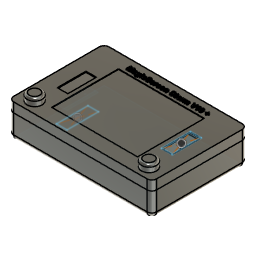
Coffret_telecran_nucleo_sharp (Autodesk Fusion 360 design; units mm, degrees)
Autodesk Fusion 360 part; units mm, degrees
(part 1 of 2)
sketch "Esquisse1" plane through (0, 0, 0) normal (0, 0, 1) x (1, 0, 0)
  line L0 (150, 100) -> (-150, 100)
  line L1 (-150, 100) -> (-150, -100)
  line L2 (-150, -100) -> (150, -100)
  line L3 (150, -100) -> (150, 100)
  line L4 (150, 100) -> (-150, -100) construction
  line L5 (-150, 100) -> (150, -100) construction
  dimension "d1" = 300
  dimension "d2" = 200
  constraint horizontal L0
  constraint perpendicular L0 L1
  constraint parallel L0 L2
  constraint parallel L1 L3
  constraint coincident L4 origin
  constraint coincident L5 origin
  measures "d1" distance of L0.start L0.end
  measures "d2" distance of L0.end L1.end
extrude "Extrusion1" add sketch "Esquisse1" along normal blind 50 makes body 1
extrude "Extrusion2" add 1 faces at (50, -33.3333, 50) along direction (0, 0, 1) blind 20 separate body on bodies 1 makes body 2
fillet "Congé1" radius 10 8 edges at (150, -100, 25) (150, 100, 25) (-150, 100, 25) (-150, -100, 25) (150, -100, 60) (150, 100, 60) (-150, 100, 60) (-150, -100, 60) on bodies 1 2
fillet "Congé2" radius 10 1 faces at (46.6667, -33.3333, 0) on bodies 1
shell "Coque1" thickness 5 removed faces 1 at (46.6667, -33.3333, 50) on bodies 1
hole "Perçage1" at (5.1249, 100, 27.601) direction (0, -1, 0) diameter 20 depth 30 tip angle 118 bodies 1
sketch "Esquisse2" plane through (0, 0, 5) normal (0, 0, 1) x (-1, 0, 0)
  line L0 (140, -90) -> (140, 90)
  line L1 (140, 90) -> (-140, 90)
  line L2 (-140, 90) -> (-140, -90)
  line L3 (-140, -90) -> (140, -90)
  line L4 (60, -50.203) -> (-60, -50.203)
  line L5 (-60, -50.203) -> (-60, 50.203)
  line L6 (-60, 50.203) -> (60, 50.203)
  line L7 (60, 50.203) -> (60, -50.203)
  line L8 (60, -50.203) -> (-60, 50.203) construction
  line L9 (-60, -50.203) -> (60, 50.203) construction
  dimension "d15" = 120
  dimension "d16" = 100.406
  constraint horizontal L4
  constraint perpendicular L4 L5
  constraint parallel L4 L6
  constraint parallel L5 L7
  constraint coincident L8 origin
  constraint coincident L9 origin
  measures "d15" distance of L4.start L4.end
  measures "d16" distance of L4.start L6.end
extrude "Extrusion3" add sketch "Esquisse2" along normal blind 35 separate body contours L4 L5 L6 L7 makes body 3
shell "Coque2" thickness 2 removed faces 1 at (-20, 16.7343, 40) on bodies 3
hole "Perçage2" at (-60, 2.6832, 20.4702) direction (1, 0, 0) diameter 20 depth 30 tip angle 118 bodies 3
hole "Perçage3" at (4.0962, 50.203, 25.4358) direction (0, -1, 0) diameter 20 depth 30 tip angle 118 bodies 3
hole "Perçage4" at (60, 1.6292, 22.5117) direction (-1, 0, 0) diameter 20 depth 3 tip angle 118 bodies 3
sketch "Esquisse3" plane through (0, 0, 5) normal (0, 0, 1) x (-1, 0, 0)
  line L0 (140, -90) -> (140, 90)
  line L1 (140, 90) -> (-140, 90)
  line L2 (-140, 90) -> (-140, -90)
  line L3 (-140, -90) -> (140, -90)
  line L4 (98, -36) -> (120, -36)
  line L5 (120, -36) -> (120, 30)
  line L6 (120, 30) -> (98, 30)
  line L7 (98, 30) -> (98, -36)
  line L8 (98, -36) -> (120, 30) construction
  line L9 (120, -36) -> (98, 30) construction
  point P0 (109, -3)
  point P1 (109, -3)
  dimension "d29" = 22
  constraint horizontal L4
  constraint perpendicular L4 L5
  constraint parallel L4 L6
  constraint parallel L5 L7
  constraint coincident L8 P1
  constraint coincident L9 P1
  measures "d29" distance of L5.end L6.end
extrude "Extrusion4" add sketch "Esquisse3" along normal blind 35 separate body contours L4 L5 L6 L7 makes body 4
hole "Perçage5" at (-109.1164, 19.6005, 40) direction (0, 0, -1) diameter 3.2 depth 3 tip angle 118 bodies 4
sketch "Esquisse4" plane through (0, 0, 40) normal (0, 0, 1) x (-1, 0, 0)
  circle A0 centre (109.1164, -19.6005) radius 1.6
  line L0 (98, 30) -> (98, -36)
  line L1 (98, -36) -> (120, -36)
  line L2 (120, -36) -> (120, 30)
  line L3 (120, 30) -> (98, 30)
hole "Perçage6" at (-109.2628, -17.4891, 40) direction (0, 0, -1) diameter 3.2 depth 3 tip angle 118 bodies 4
copy_body "Copier/Coller des corps2" bodies 4 makes body 5
move_body "Déplacer2" bodies 5 to x (1, 0, 0) y (0, 1, 0) z (0, 0, 1) at (220, 0, 0)
sketch "Esquisse5" plane through (0, 0, 70) normal (0, 0, 1) x (-1, 0, 0)
  arc A0 (150, 90) -> (140, 100) centre (140, 90) ccw
  line L0 (140, 100) -> (-140, 100)
  arc A1 (-140, 100) -> (-150, 90) centre (-140, 90) ccw
  line L1 (-150, 90) -> (-150, -90)
  arc A2 (-150, -90) -> (-140, -100) centre (-140, -90) ccw
  line L2 (-140, -100) -> (140, -100)
  arc A3 (140, -100) -> (150, -90) centre (140, -90) ccw
  line L3 (150, -90) -> (150, 90)
  line L4 (119.4908, 29.5506) -> (97.4908, 29.5506)
  line L5 (97.4908, 29.5506) -> (97.4908, -30.4494)
  line L6 (97.4908, -30.4494) -> (119.4908, -30.4494)
  line L7 (119.4908, -30.4494) -> (119.4908, 29.5506)
  line L8 (119.4908, 29.5506) -> (97.4908, -30.4494) construction
  line L9 (97.4908, 29.5506) -> (119.4908, -30.4494) construction
  point P0 (108.4908, -0.4494)
  dimension "d45" = 60
  dimension "d46" = 22
  constraint horizontal L4
  constraint perpendicular L4 L5
  constraint parallel L4 L6
  constraint parallel L5 L7
  constraint coincident L8 P0
  constraint coincident L9 P0
  measures "d45" distance of L4.end L5.end
  measures "d46" distance of L5.end L6.end
shell "Coque3" thickness 2 removed faces 1 at (46.6667, -33.3333, 50) on bodies 2
extrude "Extrusion5" cut sketch "Esquisse5" along normal blind 10 contours L4 L5 L6 L7 bodies 2
sketch "Esquisse6" plane through (0, 0, 70) normal (0, 0, 1) x (-1, 0, 0)
  line L0 (-100.2184, 29.3056) -> (-122.2184, 29.3056)
  line L1 (-122.2184, 29.3056) -> (-122.2184, -30.8073)
  line L2 (-122.2184, -30.8073) -> (-100.2184, -30.8073)
  line L3 (-100.2184, -30.8073) -> (-100.2184, 29.3056)
  line L4 (-100.2184, 29.3056) -> (-122.2184, -30.8073) construction
  line L5 (-122.2184, 29.3056) -> (-100.2184, -30.8073) construction
  point P0 (-111.2184, -0.7508)
  dimension "d51" = 60.1129
  dimension "d52" = 22
  constraint horizontal L0
  constraint perpendicular L0 L1
  constraint parallel L0 L2
  constraint parallel L1 L3
  constraint coincident L4 P0
  constraint coincident L5 P0
  measures "d51" distance of L0.end L1.end
  measures "d52" distance of L1.end L2.end
extrude "Extrusion6" cut sketch "Esquisse6" along normal blind 10 bodies 2
sketch "Esquisse7" plane through (0, 0, 70) normal (0, 0, 1) x (-1, 0, 0)
  arc A0 (150, 90) -> (140, 100) centre (140, 90) ccw
  line L0 (140, 100) -> (-140, 100)
  arc A1 (-140, 100) -> (-150, 90) centre (-140, 90) ccw
  line L1 (-150, 90) -> (-150, -90)
  arc A2 (-150, -90) -> (-140, -100) centre (-140, -90) ccw
  line L2 (-140, -100) -> (140, -100)
  arc A3 (140, -100) -> (150, -90) centre (140, -90) ccw
  line L3 (150, -90) -> (150, 90)
  line L4 (86.8869, -41.1186) -> (-95.6253, -41.0435) construction
  line L5 (-95.6253, -41.0435) -> (-95.6437, -85.9278) construction
  line L6 (-95.6437, -85.9278) -> (86.8684, -86.0029) construction
  line L7 (86.8684, -86.0029) -> (86.8869, -41.1186) construction
  dimension "d55" = 10
  text T0 "MagicScreen Storm V10 +" font "Arial" height 10 bold align centre top in box 182.5122 x 44.8843 at (86.8869, -41.1186) x (-1, 0.000412) y (-0.000412, -1) spacing 1
sketch "Esquisse8" plane through (0, 0, 70) normal (0, 0, 1) x (-1, 0, 0)
  line L0 (90, -70) -> (-90, -70)
  line L1 (-90, -70) -> (-90, 70)
  line L2 (-90, 70) -> (90, 70)
  line L3 (90, 70) -> (90, -70)
  constraint horizontal L0
  constraint vertical L1
  constraint horizontal L2
  constraint vertical L3
extrude "Extrusion7" cut sketch "Esquisse8" against normal blind 1 bodies 2
sketch "Esquisse9" plane through (0, 0, 70) normal (0, 0, 1) x (-1, 0, 0)
  circle A0 centre (120.2726, 75.6782) radius 15.6949
extrude "Extrusion8" add sketch "Esquisse9" along normal blind 15 separate body makes body 6
fillet "Congé3" radius 5 1 edges at (-105.6398, -70.0027, 85) on bodies 6
copy_body "Copier/Coller des corps3" bodies 6 makes body 7
move_body "Déplacer3" bodies 7 to x (1, 0, 0) y (0, 1, 0) z (0, 0, 1) at (240, 0, 0)
extrude "Extrusion9" add sketch "Esquisse7" along normal blind 2 text T0 bodies 2
sketch "Esquisse10" plane through (0, 0, 50) normal (0, 0, 1) x (-1, 0, 0)
  arc A0 (145, 90) -> (140, 95) centre (140, 90) ccw
  line L0 (145, 90) -> (145, -90)
  arc A1 (140, -95) -> (145, -90) centre (140, -90) ccw
  line L1 (140, -95) -> (-140, -95)
  arc A2 (-145, -90) -> (-140, -95) centre (-140, -90) ccw
  line L2 (-145, -90) -> (-145, 90)
  arc A3 (-140, 95) -> (-145, 90) centre (-140, 90) ccw
  line L3 (-140, 95) -> (140, 95)
  arc A4 (150, 90) -> (140, 100) centre (140, 90) ccw
  line L4 (140, 100) -> (-140, 100)
  arc A5 (-140, 100) -> (-150, 90) centre (-140, 90) ccw
  line L5 (-150, 90) -> (-150, -90)
  arc A6 (-150, -90) -> (-140, -100) centre (-140, -90) ccw
  line L6 (-140, -100) -> (140, -100)
  arc A7 (140, -100) -> (150, -90) centre (140, -90) ccw
  line L7 (150, -90) -> (150, 90)
  arc A8 (148, 90) -> (140, 98) centre (140, 90) ccw
  line L8 (140, 98) -> (-140, 98)
  arc A9 (-140, 98) -> (-148, 90) centre (-140, 90) ccw
  line L9 (-148, 90) -> (-148, -90)
  arc A10 (-148, -90) -> (-140, -98) centre (-140, -90) ccw
  line L10 (-140, -98) -> (140, -98)
  arc A11 (140, -98) -> (148, -90) centre (140, -90) ccw
  line L11 (148, -90) -> (148, 90)
  arc A12 (150, 90) -> (140, 100) centre (140, 90) ccw
  line L12 (150, 90) -> (150, -90)
  arc A13 (140, -100) -> (150, -90) centre (140, -90) ccw
  line L13 (140, -100) -> (-140, -100)
  arc A14 (-150, -90) -> (-140, -100) centre (-140, -90) ccw
  line L14 (-150, -90) -> (-150, 90)
  arc A15 (-140, 100) -> (-150, 90) centre (-140, 90) ccw
  line L15 (-140, 100) -> (140, 100)
extrude "Extrusion10" add sketch "Esquisse10" along normal blind 5 contours A8 L8 A9 L9 A10 L10 A11 L11 bodies 1
extrude "Extrusion12" cut sketch "Esquisse6" against normal blind 2 bodies 2
sketch "Esquisse11" plane through (0, 0, 70) normal (0, 0, 1) x (-1, 0, 0)
  line L0 (-122.2184, 29.3056) -> (-100.2184, 29.3056)
  line L1 (-100.2184, 29.3056) -> (-100.2184, -30.8073)
  line L2 (-100.2184, -30.8073) -> (-122.2184, -30.8073)
  line L3 (-122.2184, -30.8073) -> (-122.2184, 29.3056)
  line L4 (80.4323, -76.0002) -> (80.4281, -86.0002)
  line L5 (80.4281, -86.0002) -> (77.4063, -85.999)
  line L6 (77.4063, -85.999) -> (75.5947, -79.177)
  line L7 (75.5947, -79.177) -> (73.7979, -85.9975)
  line L8 (73.7979, -85.9975) -> (70.7692, -85.9963)
  line L9 (70.7692, -85.9963) -> (70.7733, -75.9963)
  line L10 (70.7733, -75.9963) -> (72.6492, -75.997)
  line L11 (72.6492, -75.997) -> (72.6459, -83.8688)
  line L12 (72.6459, -83.8688) -> (74.6342, -75.9979)
  line L13 (74.6342, -75.9979) -> (76.5782, -75.9987)
  line L14 (76.5782, -75.9987) -> (78.5532, -83.8712)
  line L15 (78.5532, -83.8712) -> (78.5564, -75.9995)
  line L16 (78.5564, -75.9995) -> (80.4323, -76.0002)
  spline S0 degree 3 poles (-73.8147, -85.9777) (-74.2685, -85.9393) (-75.1517, -85.8646) (-75.7802, -85.2424) (-76.0858, -84.9399) knots 0 0 0 0 0.132005 0.256886 0.256886 0.256886 0.256886
  spline S1 degree 3 poles (-76.0858, -84.9399) (-76.3683, -84.4062) (-77.0383, -83.1405) (-77.0518, -81.7002) (-77.0595, -80.8672) knots 0 0 0 0 0.178847 0.424093 0.424093 0.424093 0.424093
  spline S2 degree 3 poles (-77.0595, -80.8672) (-77.0502, -80.0349) (-77.0341, -78.5918) (-76.3606, -77.3247) (-76.0756, -76.7885) knots 0 0 0 0 0.245094 0.424928 0.424928 0.424928 0.424928
  spline S3 degree 3 poles (-76.0756, -76.7885) (-75.7711, -76.4903) (-75.1425, -75.8747) (-74.2636, -75.8031) (-73.8105, -75.7662) knots 0 0 0 0 0.123844 0.255615 0.255615 0.255615 0.255615
  spline S4 degree 3 poles (-73.8105, -75.7662) (-73.3484, -75.812) (-72.4293, -75.9029) (-71.7803, -76.5595) (-71.4576, -76.8859) knots 0 0 0 0 0.134755 0.268001 0.268001 0.268001 0.268001
  spline S5 degree 3 poles (-71.4576, -76.8859) (-71.1992, -77.3983) (-70.5687, -78.6489) (-70.5668, -80.0584) (-70.5657, -80.8903) knots 0 0 0 0 0.170134 0.415186 0.415186 0.415186 0.415186
  spline S6 degree 3 poles (-70.5657, -80.8903) (-70.5753, -81.7193) (-70.5919, -83.1578) (-71.2645, -84.4204) (-71.5496, -84.9554) knots 0 0 0 0 0.244076 0.423599 0.423599 0.423599 0.423599
  spline S7 degree 3 poles (-71.5496, -84.9554) (-71.8541, -85.2537) (-72.4827, -85.8692) (-73.3616, -85.9408) (-73.8147, -85.9777) knots 0 0 0 0 0.123844 0.255614 0.255614 0.255614 0.255614
  line L17 (-67.7055, -75.9393) -> (-65.7887, -75.9401)
  line L18 (-65.7887, -75.9401) -> (-65.7917, -83.1638)
  spline S8 degree 3 poles (-65.7917, -83.1638) (-65.4232, -82.857) (-64.6779, -82.2365) (-63.7726, -81.888) (-63.315, -81.7119) knots 0 0 0 0 0.142804 0.288822 0.288822 0.288822 0.288822
  line L19 (-63.315, -81.7119) -> (-63.3157, -83.4513)
  spline S9 degree 3 poles (-63.3157, -83.4513) (-63.582, -83.5598) (-64.1655, -83.7975) (-64.6714, -84.1738) (-64.9464, -84.3783) knots 0 0 0 0 0.085937 0.188242 0.188242 0.188242 0.188242
  spline S10 degree 3 poles (-64.9464, -84.3783) (-65.2145, -84.6112) (-65.7315, -85.0601) (-66.017, -85.6816) (-66.1544, -85.9808) knots 0 0 0 0 0.10515 0.202747 0.202747 0.202747 0.202747
  line L20 (-66.1544, -85.9808) -> (-67.7097, -85.9802)
  line L21 (-67.7097, -85.9802) -> (-67.7055, -75.9393)
  line L22 (-37.4493, -83.1959) -> (-39.216, -83.1952)
  line L23 (-39.216, -83.1952) -> (-39.2156, -82.2061)
  spline S11 degree 3 poles (-39.2156, -82.2061) (-39.538, -82.5421) (-40.1593, -83.1895) (-41.0469, -83.3033) (-41.4739, -83.358) knots 0 0 0 0 0.135133 0.260423 0.260423 0.260423 0.260423
  spline S12 degree 3 poles (-41.4739, -83.358) (-41.6939, -83.3482) (-42.1151, -83.3296) (-42.4982, -83.1546) (-42.6812, -83.071) knots 0 0 0 0 0.065366 0.125127 0.125127 0.125127 0.125127
  spline S13 degree 3 poles (-42.6812, -83.071) (-42.8457, -82.9601) (-43.1861, -82.7307) (-43.4061, -82.3837) (-43.5198, -82.2043) knots 0 0 0 0 0.05884 0.121768 0.121768 0.121768 0.121768
  spline S14 degree 3 poles (-43.5198, -82.2043) (-43.6773, -82.3827) (-43.9777, -82.7231) (-44.3656, -82.9583) (-44.5502, -83.0702) knots 0 0 0 0 0.070907 0.13528 0.13528 0.13528 0.13528
  spline S15 degree 3 poles (-44.5502, -83.0702) (-44.7377, -83.1537) (-45.1137, -83.321) (-45.5245, -83.3445) (-45.7304, -83.3562) knots 0 0 0 0 0.061035 0.122336 0.122336 0.122336 0.122336
  spline S16 degree 3 poles (-45.7304, -83.3562) (-45.9802, -83.3459) (-46.4529, -83.3263) (-46.8797, -83.1237) (-47.0809, -83.0283) knots 0 0 0 0 0.074123 0.140244 0.140244 0.140244 0.140244
  spline S17 degree 3 poles (-47.0809, -83.0283) (-47.2541, -82.9066) (-47.6073, -82.6588) (-47.8051, -82.2752) (-47.9059, -82.0798) knots 0 0 0 0 0.062513 0.127389 0.127389 0.127389 0.127389
  spline S18 degree 3 poles (-47.9059, -82.0798) (-47.963, -81.8785) (-48.1021, -81.3891) (-48.1027, -80.8792) (-48.103, -80.579) knots 0 0 0 0 0.062496 0.151991 0.151991 0.151991 0.151991
  line L24 (-48.103, -80.579) -> (-48.1011, -75.9473)
  line L25 (-48.1011, -75.9473) -> (-46.1844, -75.9481)
  line L26 (-46.1844, -75.9481) -> (-46.1861, -80.0886)
  spline S19 degree 3 poles (-46.1861, -80.0886) (-46.1907, -80.3879) (-46.1982, -80.8643) (-46.0456, -81.3133) (-45.9888, -81.4803) knots 0 0 0 0 0.088815 0.141427 0.141427 0.141427 0.141427
  spline S20 degree 3 poles (-45.9888, -81.4803) (-45.885, -81.5996) (-45.6694, -81.8476) (-45.3409, -81.8755) (-45.1704, -81.8899) knots 0 0 0 0 0.045633 0.094799 0.094799 0.094799 0.094799
  spline S21 degree 3 poles (-45.1704, -81.8899) (-45.0372, -81.879) (-44.7657, -81.8567) (-44.5321, -81.7162) (-44.4132, -81.6446) knots 0 0 0 0 0.039532 0.080561 0.080561 0.080561 0.080561
  spline S22 degree 3 poles (-44.4132, -81.6446) (-44.3022, -81.5501) (-44.0706, -81.3529) (-43.9593, -81.0694) (-43.9013, -80.9218) knots 0 0 0 0 0.043049 0.0898 0.0898 0.0898 0.0898
  spline S23 degree 3 poles (-43.9013, -80.9218) (-43.8558, -80.7196) (-43.7453, -80.2285) (-43.7443, -79.7245) (-43.7438, -79.428) knots 0 0 0 0 0.062007 0.1506 0.1506 0.1506 0.1506
  line L27 (-43.7438, -79.428) -> (-43.7423, -75.9491)
  line L28 (-43.7423, -75.9491) -> (-41.8256, -75.9499)
  line L29 (-41.8256, -75.9499) -> (-41.8272, -79.9199)
  spline S24 degree 3 poles (-41.8272, -79.9199) (-41.8302, -80.2109) (-41.8349, -80.6692) (-41.7547, -81.1197) (-41.7254, -81.2842) knots 0 0 0 0 0.087009 0.137055 0.137055 0.137055 0.137055
  spline S25 degree 3 poles (-41.7254, -81.2842) (-41.6887, -81.3785) (-41.619, -81.5573) (-41.4737, -81.6823) (-41.405, -81.7414) knots 0 0 0 0 0.02982 0.05659 0.05659 0.05659 0.05659
  spline S26 degree 3 poles (-41.405, -81.7414) (-41.3232, -81.7851) (-41.1426, -81.8815) (-40.9374, -81.8881) (-40.8253, -81.8917) knots 0 0 0 0 0.027479 0.060605 0.060605 0.060605 0.060605
  spline S27 degree 3 poles (-40.8253, -81.8917) (-40.6818, -81.8822) (-40.3975, -81.8634) (-40.1498, -81.7228) (-40.0271, -81.6533) knots 0 0 0 0 0.042542 0.084266 0.084266 0.084266 0.084266
  spline S28 degree 3 poles (-40.0271, -81.6533) (-39.9164, -81.5628) (-39.6882, -81.3765) (-39.574, -81.1045) (-39.5152, -80.9645) knots 0 0 0 0 0.042216 0.086988 0.086988 0.086988 0.086988
  spline S29 degree 3 poles (-39.5152, -80.9645) (-39.4717, -80.7657) (-39.3643, -80.2743) (-39.3645, -79.7706) (-39.3645, -79.4707) knots 0 0 0 0 0.060906 0.150514 0.150514 0.150514 0.150514
  line L30 (-39.3645, -79.4707) -> (-39.3631, -75.9509)
  line L31 (-39.3631, -75.9509) -> (-37.4463, -75.9517)
  line L32 (-37.4463, -75.9517) -> (-37.4493, -83.1959)
  line L33 (6.3386, -78.2753) -> (4.4287, -77.954)
  spline S30 degree 3 poles (4.4287, -77.954) (4.5643, -77.6283) (4.8259, -77.0001) (5.3456, -76.5623) (5.5958, -76.3514) knots 0 0 0 0 0.104107 0.20082 0.20082 0.20082 0.20082
  spline S31 degree 3 poles (5.5958, -76.3514) (5.8868, -76.1925) (6.5043, -75.8553) (7.2086, -75.8234) (7.581, -75.8065) knots 0 0 0 0 0.098131 0.208289 0.208289 0.208289 0.208289
  spline S32 degree 3 poles (7.581, -75.8065) (8.1591, -75.8443) (9.2481, -75.9155) (10.0166, -76.6825) (10.3773, -77.0424) knots 0 0 0 0 0.167266 0.315131 0.315131 0.315131 0.315131
  spline S33 degree 3 poles (10.3773, -77.0424) (10.5858, -77.4065) (11.0279, -78.1785) (11.0702, -79.0689) (11.0925, -79.5392) knots 0 0 0 0 0.124098 0.263046 0.263046 0.263046 0.263046
  spline S34 degree 3 poles (11.0925, -79.5392) (11.0657, -80.0923) (11.0158, -81.1238) (10.4243, -81.9656) (10.15, -82.356) knots 0 0 0 0 0.162187 0.302492 0.302492 0.302492 0.302492
  spline S35 degree 3 poles (10.15, -82.356) (9.813, -82.6543) (9.1324, -83.2568) (8.2264, -83.3375) (7.7689, -83.3783) knots 0 0 0 0 0.131335 0.26528 0.26528 0.26528 0.26528
  spline S36 degree 3 poles (7.7689, -83.3783) (7.2647, -83.3404) (6.2922, -83.2673) (5.5673, -82.6186) (5.2182, -82.3063) knots 0 0 0 0 0.147069 0.28368 0.28368 0.28368 0.28368
  spline S37 degree 3 poles (5.2182, -82.3063) (4.9492, -81.8681) (4.3378, -80.8722) (4.3302, -79.6968) (4.326, -79.0385) knots 0 0 0 0 0.151544 0.344463 0.344463 0.344463 0.344463
  line L34 (4.326, -79.0385) -> (9.1281, -79.0405)
  spline S38 degree 3 poles (9.1281, -79.0405) (9.1099, -78.7789) (9.076, -78.2916) (8.795, -77.8942) (8.6648, -77.7101) knots 0 0 0 0 0.076929 0.14329 0.14329 0.14329 0.14329
  spline S39 degree 3 poles (8.6648, -77.7101) (8.5073, -77.5728) (8.1901, -77.2963) (7.771, -77.2582) (7.56, -77.239) knots 0 0 0 0 0.061039 0.122877 0.122877 0.122877 0.122877
  spline S40 degree 3 poles (7.56, -77.239) (7.4179, -77.2476) (7.1439, -77.2641) (6.9136, -77.4127) (6.8027, -77.4843) knots 0 0 0 0 0.041891 0.080804 0.080804 0.080804 0.080804
  spline S41 degree 3 poles (6.8027, -77.4843) (6.7046, -77.5861) (6.4873, -77.8117) (6.3912, -78.1111) (6.3386, -78.2753) knots 0 0 0 0 0.041878 0.092802 0.092802 0.092802 0.092802
  line L35 (67.347, -81.029) -> (69.0863, -81.3435)
  spline S42 degree 3 poles (69.0863, -81.3435) (68.9786, -81.665) (68.7754, -82.2721) (68.2998, -82.698) (68.0761, -82.8983) knots 0 0 0 0 0.099736 0.188272 0.188272 0.188272 0.188272
  spline S43 degree 3 poles (68.0761, -82.8983) (67.7846, -83.0448) (67.118, -83.3798) (66.369, -83.3941) (65.9476, -83.4022) knots 0 0 0 0 0.096734 0.221181 0.221181 0.221181 0.221181
  spline S44 degree 3 poles (65.9476, -83.4022) (65.5707, -83.3992) (64.9168, -83.394) (64.2993, -83.1836) (64.0378, -83.0945) knots 0 0 0 0 0.112132 0.19454 0.19454 0.19454 0.19454
  spline S45 degree 3 poles (64.0378, -83.0945) (63.8479, -82.9935) (63.4932, -82.8051) (63.2644, -82.4761) (63.1582, -82.3233) knots 0 0 0 0 0.063435 0.118485 0.118485 0.118485 0.118485
  spline S46 degree 3 poles (63.1582, -82.3233) (63.0834, -82.105) (62.8942, -81.5523) (62.8976, -80.9659) (62.8997, -80.611) knots 0 0 0 0 0.0688 0.174217 0.174217 0.174217 0.174217
  line L36 (62.8997, -80.611) -> (62.9211, -78.3737)
  spline S47 degree 3 poles (62.9211, -78.3737) (62.9208, -78.0963) (62.9205, -77.6236) (62.8586, -77.1552) (62.833, -76.9616) knots 0 0 0 0 0.083079 0.141609 0.141609 0.141609 0.141609
  spline S48 degree 3 poles (62.833, -76.9616) (62.7925, -76.8043) (62.7067, -76.4707) (62.5619, -76.1581) (62.4855, -75.9929) knots 0 0 0 0 0.048629 0.103109 0.103109 0.103109 0.103109
  line L37 (62.4855, -75.9929) -> (64.3818, -75.9936)
  spline S49 degree 3 poles (64.3818, -75.9936) (64.4103, -76.0724) (64.4779, -76.2591) (64.5336, -76.4497) (64.5657, -76.5599) knots 0 0 0 0 0.025134 0.05955 0.05955 0.05955 0.05955
  spline S50 degree 3 poles (64.5657, -76.5599) (64.5789, -76.6072) (64.5998, -76.6828) (64.6246, -76.7572) (64.6339, -76.785) knots 0 0 0 0 0.014734 0.023524 0.023524 0.023524 0.023524
  spline S51 degree 3 poles (64.6339, -76.785) (64.7975, -76.6372) (65.115, -76.3502) (65.4986, -76.161) (65.6846, -76.0692) knots 0 0 0 0 0.065788 0.127687 0.127687 0.127687 0.127687
  spline S52 degree 3 poles (65.6846, -76.0692) (65.8754, -75.9997) (66.261, -75.859) (66.6711, -75.8404) (66.8784, -75.831) knots 0 0 0 0 0.06052 0.122371 0.122371 0.122371 0.122371
  spline S53 degree 3 poles (66.8784, -75.831) (67.2237, -75.8493) (67.8728, -75.8837) (68.3987, -76.2618) (68.6449, -76.4388) knots 0 0 0 0 0.101246 0.19033 0.19033 0.19033 0.19033
  spline S54 degree 3 poles (68.6449, -76.4388) (68.8318, -76.6567) (69.211, -77.0987) (69.2604, -77.6794) (69.2855, -77.9738) knots 0 0 0 0 0.083879 0.170136 0.170136 0.170136 0.170136
  spline S55 degree 3 poles (69.2855, -77.9738) (69.2744, -78.1708) (69.2528, -78.5553) (69.0773, -78.8979) (68.9917, -79.0651) knots 0 0 0 0 0.058443 0.114132 0.114132 0.114132 0.114132
  spline S56 degree 3 poles (68.9917, -79.0651) (68.8836, -79.2172) (68.6656, -79.5236) (68.3379, -79.7084) (68.1729, -79.8015) knots 0 0 0 0 0.055242 0.111336 0.111336 0.111336 0.111336
  spline S57 degree 3 poles (68.1729, -79.8015) (67.9586, -79.8881) (67.4644, -80.0879) (66.9412, -80.1921) (66.6447, -80.2511) knots 0 0 0 0 0.069179 0.1596 0.1596 0.1596 0.1596
  spline S58 degree 3 poles (66.6447, -80.2511) (66.2628, -80.3217) (65.6315, -80.4386) (65.0227, -80.641) (64.7823, -80.721) knots 0 0 0 0 0.116329 0.192272 0.192272 0.192272 0.192272
  line L38 (64.7823, -80.721) -> (64.7822, -80.9119)
  spline S59 degree 3 poles (64.7822, -80.9119) (64.7868, -81.0763) (64.7949, -81.369) (64.9755, -81.5966) (65.0547, -81.6965) knots 0 0 0 0 0.047727 0.085046 0.085046 0.085046 0.085046
  spline S60 degree 3 poles (65.0547, -81.6965) (65.1835, -81.7656) (65.5025, -81.9366) (65.8672, -81.936) (66.0847, -81.9357) knots 0 0 0 0 0.043272 0.107159 0.107159 0.107159 0.107159
  spline S61 degree 3 poles (66.0847, -81.9357) (66.2398, -81.9312) (66.5222, -81.9229) (66.7708, -81.7909) (66.8828, -81.7314) knots 0 0 0 0 0.045819 0.083375 0.083375 0.083375 0.083375
  spline S62 degree 3 poles (66.8828, -81.7314) (66.9764, -81.6448) (67.1875, -81.4494) (67.2899, -81.1793) (67.347, -81.029) knots 0 0 0 0 0.037759 0.085202 0.085202 0.085202 0.085202
  line L39 (-90, -70) -> (-90, 70)
  line L40 (-90, 70) -> (90, 70)
  line L41 (90, 70) -> (90, -70)
  line L42 (90, -70) -> (-90, -70)
  arc A0 (150, 90) -> (140, 100) centre (140, 90) ccw
  line L43 (140, 100) -> (-140, 100)
  arc A1 (-140, 100) -> (-150, 90) centre (-140, 90) ccw
  line L44 (-150, 90) -> (-150, -90)
  arc A2 (-150, -90) -> (-140, -100) centre (-140, -90) ccw
  line L45 (-140, -100) -> (140, -100)
  arc A3 (140, -100) -> (150, -90) centre (140, -90) ccw
  line L46 (150, -90) -> (150, 90)
  line L47 (52.4753, -84.2152) -> (52.4745, -85.9887)
  line L48 (52.4745, -85.9887) -> (50.5578, -85.9879)
  line L49 (50.5578, -85.9879) -> (50.5585, -84.2144)
  line L50 (50.5585, -84.2144) -> (52.4753, -84.2152)
  line L51 (42.2787, -81.0869) -> (44.1684, -80.7466)
  spline S63 degree 3 poles (44.1684, -80.7466) (44.2059, -80.9197) (44.2762, -81.2436) (44.5003, -81.4864) (44.6046, -81.5994) knots 0 0 0 0 0.052046 0.09735 0.09735 0.09735 0.09735
  spline S64 degree 3 poles (44.6046, -81.5994) (44.729, -81.683) (44.9924, -81.8598) (45.31, -81.8771) (45.4776, -81.8863) knots 0 0 0 0 0.044125 0.093421 0.093421 0.093421 0.093421
  spline S65 degree 3 poles (45.4776, -81.8863) (45.7026, -81.8677) (46.1417, -81.8315) (46.4657, -81.5339) (46.6238, -81.3888) knots 0 0 0 0 0.065652 0.128169 0.128169 0.128169 0.128169
  spline S66 degree 3 poles (46.6238, -81.3888) (46.7465, -81.1742) (47.0368, -80.6666) (47.0435, -80.078) (47.0474, -79.7382) knots 0 0 0 0 0.073069 0.17288 0.17288 0.17288 0.17288
  spline S67 degree 3 poles (47.0474, -79.7382) (47.0451, -79.3627) (47.0412, -78.7188) (46.7428, -78.1527) (46.6184, -77.9168) knots 0 0 0 0 0.110517 0.189525 0.189525 0.189525 0.189525
  spline S68 degree 3 poles (46.6184, -77.9168) (46.4587, -77.7615) (46.1338, -77.4457) (45.6819, -77.4049) (45.4522, -77.3842) knots 0 0 0 0 0.064748 0.131737 0.131737 0.131737 0.131737
  spline S69 degree 3 poles (45.4522, -77.3842) (45.2814, -77.3945) (44.9544, -77.4142) (44.6864, -77.6014) (44.5584, -77.6908) knots 0 0 0 0 0.050215 0.096136 0.096136 0.096136 0.096136
  spline S70 degree 3 poles (44.5584, -77.6908) (44.4488, -77.8271) (44.1963, -78.1411) (44.1136, -78.5373) (44.0669, -78.7615) knots 0 0 0 0 0.051803 0.119295 0.119295 0.119295 0.119295
  line L52 (44.0669, -78.7615) -> (42.1843, -78.4402)
  spline S71 degree 3 poles (42.1843, -78.4402) (42.2954, -78.0424) (42.5049, -77.2921) (43.0531, -76.7416) (43.3106, -76.4829) knots 0 0 0 0 0.121532 0.229203 0.229203 0.229203 0.229203
  spline S72 degree 3 poles (43.3106, -76.4829) (43.6268, -76.2903) (44.3098, -75.8744) (45.1111, -75.8404) (45.5415, -75.8222) knots 0 0 0 0 0.10929 0.236056 0.236056 0.236056 0.236056
  spline S73 degree 3 poles (45.5415, -75.8222) (46.0376, -75.8571) (46.9918, -75.9242) (47.7261, -76.5335) (48.0786, -76.8259) knots 0 0 0 0 0.145088 0.279038 0.279038 0.279038 0.279038
  spline S74 degree 3 poles (48.0786, -76.8259) (48.3526, -77.2108) (48.9421, -78.0386) (48.9921, -79.0574) (49.0188, -79.6026) knots 0 0 0 0 0.138834 0.298659 0.298659 0.298659 0.298659
  spline S75 degree 3 poles (49.0188, -79.6026) (48.9921, -80.1528) (48.9423, -81.1777) (48.3458, -82.0077) (48.0695, -82.3921) knots 0 0 0 0 0.1612 0.300295 0.300295 0.300295 0.300295
  spline S76 degree 3 poles (48.0695, -82.3921) (47.7143, -82.6843) (46.9708, -83.2959) (46.0075, -83.3602) (45.5043, -83.3938) knots 0 0 0 0 0.134515 0.281618 0.281618 0.281618 0.281618
  spline S77 degree 3 poles (45.5043, -83.3938) (45.0991, -83.3789) (44.3518, -83.3514) (43.7014, -82.9869) (43.4035, -82.8199) knots 0 0 0 0 0.119552 0.220555 0.220555 0.220555 0.220555
  spline S78 degree 3 poles (43.4035, -82.8199) (43.1577, -82.5953) (42.6336, -82.1166) (42.4018, -81.4439) (42.2787, -81.0869) knots 0 0 0 0 0.098323 0.209554 0.209554 0.209554 0.209554
  line L53 (25.1914, -81.0798) -> (27.0811, -80.7395)
  spline S79 degree 3 poles (27.0811, -80.7395) (27.1186, -80.9127) (27.1889, -81.2366) (27.413, -81.4794) (27.5173, -81.5924) knots 0 0 0 0 0.052046 0.09735 0.09735 0.09735 0.09735
  spline S80 degree 3 poles (27.5173, -81.5924) (27.6417, -81.6759) (27.9051, -81.8528) (28.2227, -81.8701) (28.3903, -81.8792) knots 0 0 0 0 0.044125 0.093421 0.093421 0.093421 0.093421
  spline S81 degree 3 poles (28.3903, -81.8792) (28.6152, -81.8607) (29.0544, -81.8245) (29.3784, -81.5269) (29.5365, -81.3818) knots 0 0 0 0 0.065652 0.128169 0.128169 0.128169 0.128169
  spline S82 degree 3 poles (29.5365, -81.3818) (29.6592, -81.1672) (29.9495, -80.6596) (29.9562, -80.071) (29.9601, -79.7312) knots 0 0 0 0 0.073069 0.17288 0.17288 0.17288 0.17288
  spline S83 degree 3 poles (29.9601, -79.7312) (29.9578, -79.3557) (29.9539, -78.7118) (29.6555, -78.1457) (29.5311, -77.9097) knots 0 0 0 0 0.110517 0.189525 0.189525 0.189525 0.189525
  spline S84 degree 3 poles (29.5311, -77.9097) (29.3714, -77.7545) (29.0465, -77.4386) (28.5946, -77.3979) (28.3648, -77.3772) knots 0 0 0 0 0.064748 0.131736 0.131736 0.131736 0.131736
  spline S85 degree 3 poles (28.3648, -77.3772) (28.194, -77.3875) (27.8671, -77.4071) (27.5991, -77.5943) (27.4711, -77.6838) knots 0 0 0 0 0.050215 0.096136 0.096136 0.096136 0.096136
  spline S86 degree 3 poles (27.4711, -77.6838) (27.3615, -77.8201) (27.109, -78.134) (27.0263, -78.5303) (26.9796, -78.7545) knots 0 0 0 0 0.051803 0.119295 0.119295 0.119295 0.119295
  line L54 (26.9796, -78.7545) -> (25.097, -78.4331)
  spline S87 degree 3 poles (25.097, -78.4331) (25.2081, -78.0353) (25.4176, -77.2851) (25.9658, -76.7345) (26.2233, -76.4759) knots 0 0 0 0 0.121532 0.229202 0.229202 0.229202 0.229202
  spline S88 degree 3 poles (26.2233, -76.4759) (26.5395, -76.2833) (27.2224, -75.8674) (28.0238, -75.8334) (28.4542, -75.8151) knots 0 0 0 0 0.10929 0.236056 0.236056 0.236056 0.236056
  spline S89 degree 3 poles (28.4542, -75.8151) (28.9503, -75.85) (29.9045, -75.9172) (30.6388, -76.5264) (30.9913, -76.8189) knots 0 0 0 0 0.145088 0.279037 0.279037 0.279037 0.279037
  spline S90 degree 3 poles (30.9913, -76.8189) (31.2653, -77.2037) (31.8548, -78.0315) (31.9047, -79.0504) (31.9315, -79.5956) knots 0 0 0 0 0.138834 0.298659 0.298659 0.298659 0.298659
  spline S91 degree 3 poles (31.9315, -79.5956) (31.9047, -80.1457) (31.855, -81.1707) (31.2585, -82.0006) (30.9822, -82.3851) knots 0 0 0 0 0.1612 0.300295 0.300295 0.300295 0.300295
  spline S92 degree 3 poles (30.9822, -82.3851) (30.627, -82.6772) (29.8835, -83.2889) (28.9201, -83.3532) (28.4169, -83.3867) knots 0 0 0 0 0.134515 0.281619 0.281619 0.281619 0.281619
  spline S93 degree 3 poles (28.4169, -83.3867) (28.0118, -83.3718) (27.2645, -83.3444) (26.6141, -82.9798) (26.3162, -82.8129) knots 0 0 0 0 0.119552 0.220555 0.220555 0.220555 0.220555
  spline S94 degree 3 poles (26.3162, -82.8129) (26.0703, -82.5883) (25.5463, -82.1096) (25.3145, -81.4369) (25.1914, -81.0798) knots 0 0 0 0 0.098323 0.209554 0.209554 0.209554 0.209554
  line L55 (14.108, -78.2785) -> (12.1982, -77.9572)
  spline S95 degree 3 poles (12.1982, -77.9572) (12.3338, -77.6315) (12.5953, -77.0033) (13.115, -76.5655) (13.3653, -76.3546) knots 0 0 0 0 0.104107 0.20082 0.20082 0.20082 0.20082
  spline S96 degree 3 poles (13.3653, -76.3546) (13.6562, -76.1957) (14.2737, -75.8585) (14.978, -75.8266) (15.3505, -75.8097) knots 0 0 0 0 0.098131 0.20829 0.20829 0.20829 0.20829
  spline S97 degree 3 poles (15.3505, -75.8097) (15.9285, -75.8475) (17.0175, -75.9187) (17.7861, -76.6857) (18.1467, -77.0456) knots 0 0 0 0 0.167266 0.31513 0.31513 0.31513 0.31513
  spline S98 degree 3 poles (18.1467, -77.0456) (18.3553, -77.4097) (18.7974, -78.1817) (18.8396, -79.0721) (18.8619, -79.5424) knots 0 0 0 0 0.124098 0.263046 0.263046 0.263046 0.263046
  spline S99 degree 3 poles (18.8619, -79.5424) (18.8351, -80.0955) (18.7852, -81.1269) (18.1937, -81.9688) (17.9194, -82.3592) knots 0 0 0 0 0.162187 0.302492 0.302492 0.302492 0.302492
  spline S100 degree 3 poles (17.9194, -82.3592) (17.5824, -82.6575) (16.9018, -83.26) (15.9958, -83.3407) (15.5384, -83.3814) knots 0 0 0 0 0.131335 0.26528 0.26528 0.26528 0.26528
  spline S101 degree 3 poles (15.5384, -83.3814) (15.0342, -83.3436) (14.0617, -83.2705) (13.3367, -82.6218) (12.9876, -82.3095) knots 0 0 0 0 0.147069 0.28368 0.28368 0.28368 0.28368
  spline S102 degree 3 poles (12.9876, -82.3095) (12.7187, -81.8713) (12.1072, -80.8754) (12.0996, -79.7) (12.0954, -79.0417) knots 0 0 0 0 0.151544 0.344463 0.344463 0.344463 0.344463
  line L56 (12.0954, -79.0417) -> (16.8976, -79.0437)
  spline S103 degree 3 poles (16.8976, -79.0437) (16.8794, -78.7821) (16.8454, -78.2948) (16.5644, -77.8974) (16.4343, -77.7133) knots 0 0 0 0 0.076929 0.14329 0.14329 0.14329 0.14329
  spline S104 degree 3 poles (16.4343, -77.7133) (16.2767, -77.576) (15.9596, -77.2995) (15.5404, -77.2614) (15.3294, -77.2422) knots 0 0 0 0 0.061038 0.122877 0.122877 0.122877 0.122877
  spline S105 degree 3 poles (15.3294, -77.2422) (15.1874, -77.2508) (14.9134, -77.2673) (14.6831, -77.4159) (14.5722, -77.4875) knots 0 0 0 0 0.041892 0.080803 0.080803 0.080803 0.080803
  spline S106 degree 3 poles (14.5722, -77.4875) (14.4741, -77.5893) (14.2567, -77.8149) (14.1607, -78.1143) (14.108, -78.2785) knots 0 0 0 0 0.041878 0.092802 0.092802 0.092802 0.092802
  line L57 (-9.153, -79.2171) -> (-11.1176, -79.4073)
  spline S107 degree 3 poles (-11.1176, -79.4073) (-11.1818, -79.1086) (-11.2993, -78.5621) (-11.6667, -78.1438) (-11.8332, -77.9541) knots 0 0 0 0 0.089859 0.164382 0.164382 0.164382 0.164382
  spline S108 degree 3 poles (-11.8332, -77.9541) (-12.04, -77.8189) (-12.484, -77.5286) (-13.0156, -77.5032) (-13.2996, -77.4896) knots 0 0 0 0 0.0728 0.156317 0.156317 0.156317 0.156317
  spline S109 degree 3 poles (-13.2996, -77.4896) (-13.5923, -77.4973) (-14.118, -77.5111) (-14.5672, -77.7794) (-14.7663, -77.8983) knots 0 0 0 0 0.086047 0.154532 0.154532 0.154532 0.154532
  spline S110 degree 3 poles (-14.7663, -77.8983) (-14.9115, -78.038) (-15.1891, -78.305) (-15.2403, -78.6853) (-15.2647, -78.8667) knots 0 0 0 0 0.058494 0.11181 0.11181 0.11181 0.11181
  spline S111 degree 3 poles (-15.2647, -78.8667) (-15.2568, -78.9793) (-15.2415, -79.1991) (-15.1151, -79.3793) (-15.0535, -79.4671) knots 0 0 0 0 0.033166 0.064726 0.064726 0.064726 0.064726
  spline S112 degree 3 poles (-15.0535, -79.4671) (-14.9629, -79.5515) (-14.7532, -79.7468) (-14.4837, -79.847) (-14.3306, -79.9039) knots 0 0 0 0 0.036813 0.085193 0.085193 0.085193 0.085193
  spline S113 degree 3 poles (-14.3306, -79.9039) (-14.1371, -79.9621) (-13.6024, -80.1227) (-13.0602, -80.256) (-12.7141, -80.3412) knots 0 0 0 0 0.0606 0.167477 0.167477 0.167477 0.167477
  spline S114 degree 3 poles (-12.7141, -80.3412) (-12.2404, -80.4617) (-11.4252, -80.6692) (-10.7282, -81.1357) (-10.4362, -81.3312) knots 0 0 0 0 0.14523 0.24996 0.24996 0.24996 0.24996
  spline S115 degree 3 poles (-10.4362, -81.3312) (-10.1678, -81.6191) (-9.6371, -82.1883) (-9.5562, -82.9617) (-9.5162, -83.3439) knots 0 0 0 0 0.114701 0.226743 0.226743 0.226743 0.226743
  spline S116 degree 3 poles (-9.5162, -83.3439) (-9.5348, -83.5952) (-9.5724, -84.1021) (-9.8211, -84.5457) (-9.9465, -84.7693) knots 0 0 0 0 0.074618 0.150525 0.150525 0.150525 0.150525
  spline S117 degree 3 poles (-9.9465, -84.7693) (-10.1112, -84.9802) (-10.4497, -85.4135) (-10.9423, -85.6591) (-11.1952, -85.7852) knots 0 0 0 0 0.07921 0.162795 0.162795 0.162795 0.162795
  spline S118 degree 3 poles (-11.1952, -85.7852) (-11.4933, -85.8864) (-12.132, -86.1033) (-12.8069, -86.1222) (-13.1667, -86.1323) knots 0 0 0 0 0.093909 0.201185 0.201185 0.201185 0.201185
  spline S119 degree 3 poles (-13.1667, -86.1323) (-13.7328, -86.1155) (-14.7532, -86.0852) (-15.6139, -85.5459) (-15.9972, -85.3057) knots 0 0 0 0 0.166191 0.299601 0.299601 0.299601 0.299601
  spline S120 degree 3 poles (-15.9972, -85.3057) (-16.2778, -85.0019) (-16.8533, -84.3788) (-16.9497, -83.5347) (-16.999, -83.102) knots 0 0 0 0 0.120771 0.247752 0.247752 0.247752 0.247752
  line L58 (-16.999, -83.102) -> (-14.9799, -83.0142)
  spline S121 degree 3 poles (-14.9799, -83.0142) (-14.9327, -83.2458) (-14.8467, -83.6674) (-14.5532, -83.979) (-14.421, -84.1195) knots 0 0 0 0 0.069259 0.126039 0.126039 0.126039 0.126039
  spline S122 degree 3 poles (-14.421, -84.1195) (-14.2483, -84.2186) (-13.8555, -84.4442) (-13.4005, -84.455) (-13.1456, -84.461) knots 0 0 0 0 0.058882 0.13389 0.13389 0.13389 0.13389
  spline S123 degree 3 poles (-13.1456, -84.461) (-12.8781, -84.4527) (-12.3895, -84.4375) (-11.9613, -84.2052) (-11.7675, -84.1001) knots 0 0 0 0 0.078964 0.144211 0.144211 0.144211 0.144211
  spline S124 degree 3 poles (-11.7675, -84.1001) (-11.674, -84.0166) (-11.4879, -83.8505) (-11.4604, -83.6027) (-11.4467, -83.4795) knots 0 0 0 0 0.03624 0.072106 0.072106 0.072106 0.072106
  spline S125 degree 3 poles (-11.4467, -83.4795) (-11.4605, -83.3644) (-11.489, -83.1273) (-11.6591, -82.9589) (-11.7466, -82.8723) knots 0 0 0 0 0.033757 0.069526 0.069526 0.069526 0.069526
  spline S126 degree 3 poles (-11.7466, -82.8723) (-11.9618, -82.7552) (-12.5438, -82.4385) (-13.1927, -82.2941) (-13.6017, -82.203) knots 0 0 0 0 0.073213 0.198018 0.198018 0.198018 0.198018
  spline S127 degree 3 poles (-13.6017, -82.203) (-14.0335, -82.0992) (-14.78, -81.9196) (-15.4816, -81.6097) (-15.7774, -81.4791) knots 0 0 0 0 0.132891 0.229702 0.229702 0.229702 0.229702
  spline S128 degree 3 poles (-15.7774, -81.4791) (-15.9998, -81.346) (-16.4386, -81.0836) (-16.7356, -80.6675) (-16.882, -80.4622) knots 0 0 0 0 0.076824 0.151588 0.151588 0.151588 0.151588
  spline S129 degree 3 poles (-16.882, -80.4622) (-16.9992, -80.2272) (-17.2483, -79.7276) (-17.2715, -79.1687) (-17.2838, -78.8727) knots 0 0 0 0 0.077881 0.165602 0.165602 0.165602 0.165602
  spline S130 degree 3 poles (-17.2838, -78.8727) (-17.2631, -78.5897) (-17.2212, -78.0184) (-16.945, -77.5164) (-16.8056, -77.2631) knots 0 0 0 0 0.084071 0.169684 0.169684 0.169684 0.169684
  spline S131 degree 3 poles (-16.8056, -77.2631) (-16.6275, -77.028) (-16.2651, -76.5496) (-15.7278, -76.2814) (-15.4546, -76.145) knots 0 0 0 0 0.087239 0.177491 0.177491 0.177491 0.177491
  spline S132 degree 3 poles (-15.4546, -76.145) (-15.1303, -76.0398) (-14.4238, -75.8108) (-13.6805, -75.7936) (-13.2784, -75.7843) knots 0 0 0 0 0.101736 0.22162 0.22162 0.22162 0.22162
  spline S133 degree 3 poles (-13.2784, -75.7843) (-12.703, -75.8051) (-11.6514, -75.843) (-10.7667, -76.4044) (-10.3661, -76.6586) knots 0 0 0 0 0.169048 0.308956 0.308956 0.308956 0.308956
  spline S134 degree 3 poles (-10.3661, -76.6586) (-10.06, -77.0011) (-9.4066, -77.7322) (-9.241, -78.7018) (-9.153, -79.2171) knots 0 0 0 0 0.135061 0.288292 0.288292 0.288292 0.288292
  spline S135 degree 3 poles (-23.1777, -79.682) (-23.1986, -79.9999) (-23.2409, -80.6451) (-23.5118, -81.2324) (-23.6491, -81.5304) knots 0 0 0 0 0.094697 0.192205 0.192205 0.192205 0.192205
  spline S136 degree 3 poles (-23.6491, -81.5304) (-23.8212, -81.8099) (-24.1625, -82.3645) (-24.7089, -82.7185) (-24.9799, -82.8941) knots 0 0 0 0 0.097119 0.192686 0.192686 0.192686 0.192686
  spline S137 degree 3 poles (-24.9799, -82.8941) (-25.2803, -83.0312) (-25.8935, -83.3111) (-26.567, -83.3461) (-26.9105, -83.364) knots 0 0 0 0 0.098143 0.20029 0.20029 0.20029 0.20029
  spline S138 degree 3 poles (-26.9105, -83.364) (-27.4289, -83.3239) (-28.4398, -83.2458) (-29.2229, -82.6044) (-29.6044, -82.2919) knots 0 0 0 0 0.151935 0.296238 0.296238 0.296238 0.296238
  spline S139 degree 3 poles (-29.6044, -82.2919) (-29.9106, -81.9072) (-30.5382, -81.1187) (-30.6146, -80.1124) (-30.6538, -79.5971) knots 0 0 0 0 0.144026 0.295199 0.295199 0.295199 0.295199
  spline S140 degree 3 poles (-30.6538, -79.5971) (-30.6133, -79.0766) (-30.534, -78.0581) (-29.899, -77.2595) (-29.5886, -76.869) knots 0 0 0 0 0.152744 0.298899 0.298899 0.298899 0.298899
  spline S141 degree 3 poles (-29.5886, -76.869) (-29.2083, -76.5549) (-28.4338, -75.915) (-27.4313, -75.8337) (-26.921, -75.7923) knots 0 0 0 0 0.144307 0.293922 0.293922 0.293922 0.293922
  spline S142 degree 3 poles (-26.921, -75.7923) (-26.5921, -75.8116) (-25.9313, -75.8502) (-25.3234, -76.1119) (-25.018, -76.2433) knots 0 0 0 0 0.098023 0.196906 0.196906 0.196906 0.196906
  spline S143 degree 3 poles (-25.018, -76.2433) (-24.7363, -76.41) (-24.176, -76.7416) (-23.823, -77.2885) (-23.6475, -77.5604) knots 0 0 0 0 0.096745 0.192416 0.192416 0.192416 0.192416
  spline S144 degree 3 poles (-23.6475, -77.5604) (-23.5105, -77.8783) (-23.219, -78.5546) (-23.192, -79.2915) (-23.1777, -79.682) knots 0 0 0 0 0.102934 0.218982 0.218982 0.218982 0.218982
  line L59 (-56.4572, -75.9439) -> (-52.887, -85.9454)
  line L60 (-52.887, -85.9454) -> (-55.0766, -85.9445)
  line L61 (-55.0766, -85.9445) -> (-57.6043, -78.5423)
  line L62 (-57.6043, -78.5423) -> (-60.0562, -85.9424)
  line L63 (-60.0562, -85.9424) -> (-62.198, -85.9415)
  line L64 (-62.198, -85.9415) -> (-58.6127, -75.943)
  line L65 (-58.6127, -75.943) -> (-56.4572, -75.9439)
  line L66 (-33.9879, -75.9532) -> (-32.0711, -75.9539)
  line L67 (-32.0711, -75.9539) -> (-32.0741, -83.1981)
  line L68 (-32.0741, -83.1981) -> (-33.8545, -83.1974)
  line L69 (-33.8545, -83.1974) -> (-33.854, -82.1674)
  spline S145 degree 3 poles (-33.854, -82.1674) (-33.9874, -82.3789) (-34.2149, -82.7396) (-34.539, -83.015) (-34.673, -83.1289) knots 0 0 0 0 0.074439 0.126933 0.126933 0.126933 0.126933
  spline S146 degree 3 poles (-34.673, -83.1289) (-34.801, -83.1964) (-35.0615, -83.3339) (-35.3557, -83.3515) (-35.5053, -83.3604) knots 0 0 0 0 0.042907 0.087284 0.087284 0.087284 0.087284
  spline S147 degree 3 poles (-35.5053, -83.3604) (-35.7235, -83.3441) (-36.1689, -83.3108) (-36.565, -83.1039) (-36.7671, -82.9984) knots 0 0 0 0 0.064923 0.132504 0.132504 0.132504 0.132504
  line L70 (-36.7671, -82.9984) -> (-36.1729, -81.3274)
  spline S148 degree 3 poles (-36.1729, -81.3274) (-36.0215, -81.4188) (-35.7427, -81.587) (-35.4201, -81.6245) (-35.2727, -81.6416) knots 0 0 0 0 0.052318 0.096337 0.096337 0.096337 0.096337
  spline S149 degree 3 poles (-35.2727, -81.6416) (-35.1452, -81.6335) (-34.8979, -81.6177) (-34.6908, -81.4823) (-34.5904, -81.4168) knots 0 0 0 0 0.0376 0.072931 0.072931 0.072931 0.072931
  spline S150 degree 3 poles (-34.5904, -81.4168) (-34.4993, -81.3183) (-34.2876, -81.0896) (-34.1978, -80.7897) (-34.1467, -80.6188) knots 0 0 0 0 0.039764 0.092363 0.092363 0.092363 0.092363
  spline S151 degree 3 poles (-34.1467, -80.6188) (-34.1015, -80.3203) (-33.9798, -79.5163) (-33.9854, -78.7023) (-33.9888, -78.1905) knots 0 0 0 0 0.090468 0.243656 0.243656 0.243656 0.243656
  line L71 (-33.9888, -78.1905) -> (-33.9879, -75.9532)
  line L72 (-22.2924, -83.2022) -> (-22.2918, -81.6742)
  line L73 (-22.2918, -81.6742) -> (-20.9821, -81.6747)
  line L74 (-20.9821, -81.6747) -> (-20.9809, -78.7552)
  spline S152 degree 3 poles (-20.9809, -78.7552) (-20.9785, -78.5208) (-20.9751, -78.1745) (-21.0049, -77.8297) (-21.0146, -77.7184) knots 0 0 0 0 0.070264 0.103786 0.103786 0.103786 0.103786
  spline S153 degree 3 poles (-21.0146, -77.7184) (-21.0323, -77.6723) (-21.0686, -77.5781) (-21.1457, -77.5129) (-21.185, -77.4796) knots 0 0 0 0 0.014569 0.029762 0.029762 0.029762 0.029762
  spline S154 degree 3 poles (-21.185, -77.4796) (-21.2338, -77.4517) (-21.3352, -77.3939) (-21.4519, -77.3873) (-21.5124, -77.3839) knots 0 0 0 0 0.016629 0.034523 0.034523 0.034523 0.034523
  spline S155 degree 3 poles (-21.5124, -77.3839) (-21.6217, -77.3957) (-21.8861, -77.4241) (-22.1365, -77.5147) (-22.2832, -77.5678) knots 0 0 0 0 0.032896 0.079499 0.079499 0.079499 0.079499
  line L75 (-22.2832, -77.5678) -> (-22.4464, -76.0807)
  spline S156 degree 3 poles (-22.4464, -76.0807) (-22.211, -75.9973) (-21.7213, -75.8237) (-21.2018, -75.8047) (-20.9319, -75.7948) knots 0 0 0 0 0.07445 0.15492 0.15492 0.15492 0.15492
  spline S157 degree 3 poles (-20.9319, -75.7948) (-20.7661, -75.8009) (-20.4462, -75.8126) (-20.1433, -75.9159) (-19.9975, -75.9657) knots 0 0 0 0 0.049468 0.09545 0.09545 0.09545 0.09545
  spline S158 degree 3 poles (-19.9975, -75.9657) (-19.871, -76.0248) (-19.6361, -76.1346) (-19.4634, -76.3273) (-19.3837, -76.4162) knots 0 0 0 0 0.041375 0.076828 0.076828 0.076828 0.076828
  spline S159 degree 3 poles (-19.3837, -76.4162) (-19.3241, -76.5233) (-19.1933, -76.758) (-19.1445, -77.0227) (-19.118, -77.1666) knots 0 0 0 0 0.036531 0.080083 0.080083 0.080083 0.080083
  spline S160 degree 3 poles (-19.118, -77.1666) (-19.1004, -77.3348) (-19.0535, -77.7835) (-19.0558, -78.235) (-19.0572, -78.5173) knots 0 0 0 0 0.050687 0.135285 0.135285 0.135285 0.135285
  line L76 (-19.0572, -78.5173) -> (-19.0585, -81.6755)
  line L77 (-19.0585, -81.6755) -> (-18.1785, -81.6759)
  line L78 (-18.1785, -81.6759) -> (-18.1792, -83.2039)
  line L79 (-18.1792, -83.2039) -> (-19.0591, -83.2035)
  line L80 (-19.0591, -83.2035) -> (-19.0597, -84.6428)
  line L81 (-19.0597, -84.6428) -> (-20.9838, -85.7607)
  line L82 (-20.9838, -85.7607) -> (-20.9827, -83.2027)
  line L83 (-20.9827, -83.2027) -> (-22.2924, -83.2022)
  line L84 (-3.8242, -75.9656) -> (-1.9074, -75.9664)
  line L85 (-1.9074, -75.9664) -> (-1.909, -79.6635)
  spline S161 degree 3 poles (-1.909, -79.6635) (-1.9125, -79.9866) (-1.9181, -80.4959) (-1.8219, -80.9953) (-1.7868, -81.1779) knots 0 0 0 0 0.09657 0.152248 0.152248 0.152248 0.152248
  spline S162 degree 3 poles (-1.7868, -81.1779) (-1.7405, -81.2865) (-1.65, -81.499) (-1.4717, -81.6454) (-1.3846, -81.7169) knots 0 0 0 0 0.03486 0.068149 0.068149 0.068149 0.068149
  spline S163 degree 3 poles (-1.3846, -81.7169) (-1.2863, -81.7726) (-1.0813, -81.8889) (-0.8457, -81.9016) (-0.723, -81.9082) knots 0 0 0 0 0.03341 0.069708 0.069708 0.069708 0.069708
  spline S164 degree 3 poles (-0.723, -81.9082) (-0.5619, -81.8973) (-0.2427, -81.8758) (0.0338, -81.7152) (0.1707, -81.6357) knots 0 0 0 0 0.047727 0.094557 0.094557 0.094557 0.094557
  spline S165 degree 3 poles (0.1707, -81.6357) (0.2923, -81.5377) (0.5347, -81.3423) (0.6562, -81.0557) (0.7167, -80.9129) knots 0 0 0 0 0.046078 0.091844 0.091844 0.091844 0.091844
  spline S166 degree 3 poles (0.7167, -80.9129) (0.7581, -80.6997) (0.8647, -80.1509) (0.8622, -79.591) (0.8607, -79.2485) knots 0 0 0 0 0.065014 0.167396 0.167396 0.167396 0.167396
  line L86 (0.8607, -79.2485) -> (0.862, -75.9675)
  line L87 (0.862, -75.9675) -> (2.7788, -75.9683)
  line L88 (2.7788, -75.9683) -> (2.7758, -83.2125)
  line L89 (2.7758, -83.2125) -> (0.9955, -83.2118)
  line L90 (0.9955, -83.2118) -> (0.9959, -82.1476)
  spline S167 degree 3 poles (0.9959, -82.1476) (0.6647, -82.5056) (0.0165, -83.2061) (-0.9294, -83.3192) (-1.3921, -83.3745) knots 0 0 0 0 0.141242 0.276424 0.276424 0.276424 0.276424
  spline S168 degree 3 poles (-1.3921, -83.3745) (-1.5966, -83.3658) (-1.9954, -83.3488) (-2.3694, -83.2098) (-2.5516, -83.1421) knots 0 0 0 0 0.060985 0.118911 0.118911 0.118911 0.118911
  spline S169 degree 3 poles (-2.5516, -83.1421) (-2.7124, -83.066) (-3.0139, -82.9233) (-3.238, -82.677) (-3.3426, -82.5619) knots 0 0 0 0 0.052756 0.098943 0.098943 0.098943 0.098943
  spline S170 degree 3 poles (-3.3426, -82.5619) (-3.4265, -82.4391) (-3.5958, -82.1914) (-3.6767, -81.9025) (-3.7174, -81.7569) knots 0 0 0 0 0.044308 0.089338 0.089338 0.089338 0.089338
  spline S171 degree 3 poles (-3.7174, -81.7569) (-3.749, -81.5748) (-3.823, -81.1485) (-3.825, -80.7156) (-3.8261, -80.4676) knots 0 0 0 0 0.05535 0.129581 0.129581 0.129581 0.129581
  line L91 (-3.8261, -80.4676) -> (-3.8242, -75.9656)
  line L92 (-84.8275, -77.3715) -> (-84.8286, -79.9704)
  line L93 (-84.8286, -79.9704) -> (-82.2092, -79.9715)
  line L94 (-82.2092, -79.9715) -> (-82.21, -81.7655)
  line L95 (-82.21, -81.7655) -> (-84.8293, -81.7644)
  line L96 (-84.8293, -81.7644) -> (-84.8304, -84.3633)
  line L97 (-84.8304, -84.3633) -> (-86.5766, -84.3626)
  line L98 (-86.5766, -84.3626) -> (-86.5756, -81.7637)
  line L99 (-86.5756, -81.7637) -> (-89.2018, -81.7626)
  line L100 (-89.2018, -81.7626) -> (-89.201, -79.9686)
  line L101 (-89.201, -79.9686) -> (-86.5748, -79.9697)
  line L102 (-86.5748, -79.9697) -> (-86.5738, -77.3708)
  line L103 (-86.5738, -77.3708) -> (-84.8275, -77.3715)
  line L104 (21.9057, -75.9762) -> (23.8224, -75.9769)
  line L105 (23.8224, -75.9769) -> (23.8195, -83.2211)
  line L106 (23.8195, -83.2211) -> (22.0391, -83.2204)
  line L107 (22.0391, -83.2204) -> (22.0395, -82.1904)
  spline S172 degree 3 poles (22.0395, -82.1904) (21.9061, -82.4019) (21.6787, -82.7626) (21.3546, -83.038) (21.2206, -83.1519) knots 0 0 0 0 0.074439 0.126933 0.126933 0.126933 0.126933
  spline S173 degree 3 poles (21.2206, -83.1519) (21.0925, -83.2194) (20.832, -83.3569) (20.5379, -83.3745) (20.3883, -83.3834) knots 0 0 0 0 0.042907 0.087284 0.087284 0.087284 0.087284
  spline S174 degree 3 poles (20.3883, -83.3834) (20.1701, -83.3671) (19.7247, -83.3338) (19.3285, -83.1269) (19.1265, -83.0214) knots 0 0 0 0 0.064923 0.132504 0.132504 0.132504 0.132504
  line L108 (19.1265, -83.0214) -> (19.7206, -81.3504)
  spline S175 degree 3 poles (19.7206, -81.3504) (19.8721, -81.4418) (20.1509, -81.61) (20.4735, -81.6475) (20.6209, -81.6646) knots 0 0 0 0 0.052317 0.096337 0.096337 0.096337 0.096337
  spline S176 degree 3 poles (20.6209, -81.6646) (20.7484, -81.6565) (20.9957, -81.6408) (21.2028, -81.5054) (21.3031, -81.4398) knots 0 0 0 0 0.0376 0.072931 0.072931 0.072931 0.072931
  spline S177 degree 3 poles (21.3031, -81.4398) (21.3943, -81.3413) (21.606, -81.1126) (21.6957, -80.8127) (21.7469, -80.6418) knots 0 0 0 0 0.039764 0.092363 0.092363 0.092363 0.092363
  spline S178 degree 3 poles (21.7469, -80.6418) (21.792, -80.3433) (21.9138, -79.5393) (21.9082, -78.7253) (21.9047, -78.2135) knots 0 0 0 0 0.090468 0.243656 0.243656 0.243656 0.243656
  line L109 (21.9047, -78.2135) -> (21.9057, -75.9762)
  line L110 (41.3245, -79.2379) -> (39.3599, -79.4281)
  spline S179 degree 3 poles (39.3599, -79.4281) (39.2957, -79.1294) (39.1781, -78.5829) (38.8108, -78.1645) (38.6443, -77.9749) knots 0 0 0 0 0.089859 0.164382 0.164382 0.164382 0.164382